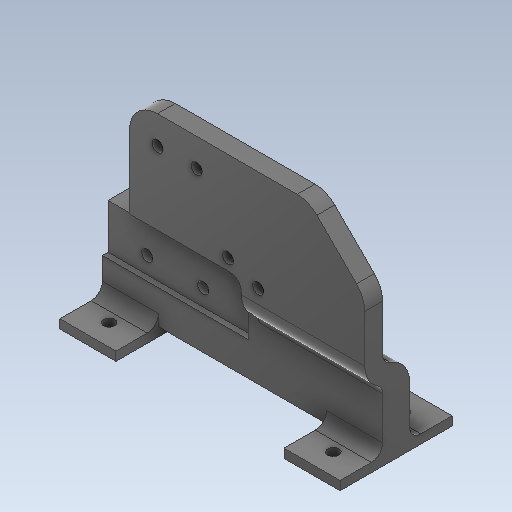
# Autodesk Inventor part: body
Saved by Autodesk Inventor 2020.3 (Build 243373000, 373)
## iProperties
Created: 2021-06-19
Part Number: body
Material: Steel, Mild
Document SubType Name: Modeling
Designer: 0x6f736f646f
Density: 7.85 g/cm^3
Appearance: Smooth - Black
Mass: 6199.14 g
Surface Area: 1192.64 cm^2
Volume: 789.699 cm^3
Author: 0x6f736f646f
Autodesk Inventor part; units mm, degrees
ref_plane "YZ Plane" through (0, 0, 0) normal (1, 0, 0) x (0, 1, 0)
sketch "Sketch1" plane through (0, 0, 0) normal (1, 0, 0) x (0, 1, 0)
  line L0 (0, 0) -> (110, 0)
  line L1 (110, 0) -> (110, -15.875)
  line L2 (110, -15.875) -> (0, -15.875)
  line L3 (0, -15.875) -> (0, -40)
  line L4 (0, -40) -> (-15.875, -40)
  line L5 (-15.875, -40) -> (-70, -40)
  line L6 (-70, -40) -> (-70, -15.875)
  line L7 (-70, -15.875) -> (-15.875, -15.875)
  line L8 (-15.875, -15.875) -> (-15.875, 0)
  line L9 (-15.875, 0) -> (0, 0)
  dimension "d1" = 15.875
  dimension "d2" = 40
  dimension "d3" = 70
  dimension "d4" = 180
  dimension "d5" = 15.875
  constraints: 20 end point, 9 perpendicular, 4 point on line, 1 horizontal
  measures "d1" distance of L0.end L1.end
  measures "d2" distance between parallel lines of L5 L0
  measures "d3" distance between parallel lines of L6 L3
  measures "d4" distance between parallel lines of L6 L1
  measures "d5" distance between parallel lines of L3 L8
extrude "Extrusion1" add sketch "Sketch1" along normal blind 250
sketch "Sketch2" plane through (250, 0, 0) normal (1, 0, 0) x (0, 0, -1)
  line L0 (15.875, -15.875) -> (15.875, -70) projected
  line L1 (15.875, -70) -> (-22.0625, -70)
  line L2 (-22.0625, -70) -> (-22.0625, -77.9375)
  line L3 (-22.0625, -77.9375) -> (77.9375, -77.9375)
  line L4 (77.9375, -77.9375) -> (77.9375, -70)
  line L5 (15.875, -70) -> (40, -70) projected
  line L6 (77.9375, -70) -> (40, -70)
  line L7 (40, -70) -> (15.875, -70)
  point P0 (0, 0)
  dimension "d8" = 100
  dimension "d9" = 7.9375
  constraints: 12 end point, 4 perpendicular, 2 collinear, 1 horizontal, 1 point on line
  measures "d8" distance of L2.end L3.end
  measures "d9" distance between parallel lines of L3 L6
extrude "Extrusion2" add sketch "Sketch2" against normal blind 50
sketch "Sketch3" plane through (250, -70, -40) normal (0, 1, 0) x (1, 0, 0)
  circle A0 centre (-25, 18.9688) radius 5
  line L0 (-50, 0) -> (-50, 37.9375) projected
  line L1 (-50, 18.9688) -> (0, 18.9688)
  line L2 (0, 37.9375) -> (0, 0) projected
  point P0 (-250, -40)
  point P1 (-25, 18.9688)
  dimension "d12" = 10
  dimension "d13" = 25
  constraints: 3 midpoint, 2 end point, 1 centre point, 1 coincident
  measures "d12" diameter of A0
  measures "d13" distance from line of L2 A0.centre
extrude "Extrusion3" cut sketch "Sketch3" against normal through all
ref_plane "Work Plane1" through (0, -70, -27.9375) normal (0, 0, 1) x (1, 0, 0)
mirror "Mirror1" about plane through (0, -70, -27.9375) normal (0, 0, 1) of "Extrusion3"
fillet "Fillet1" radius 10 2 edges at (225, -70, -40) (225, -70, -15.875)
ref_plane "Work Plane2" through (125, 0, 0) normal (1, 0, 0) x (0, 0, -1)
mirror "Mirror2" about plane through (125, 0, 0) normal (1, 0, 0) of "Extrusion2", "Extrusion3", "Mirror1", "Fillet1"
sketch "Sketch6" plane through (0, 0, -15.875) normal (0, 0, -1) x (-1, 0, 0)
  line L0 (0, 0) -> (-250, 0) projected
  line L1 (0, 0) -> (-140, 0)
  line L2 (-140, 0) -> (-140, 20)
  line L3 (-140, 20) -> (-40, 20)
  line L4 (-40, 20) -> (-40, 110)
  line L5 (0, 110) -> (-250, 110) projected
  line L6 (-40, 110) -> (0, 110)
  line L7 (0, 0) -> (0, 110) projected
  line L8 (0, 110) -> (0, 0)
  line L9 (-250, 110) -> (-250, 60)
  line L10 (-250, 0) -> (-250, 110) projected
  line L11 (-250, 60) -> (-200, 110)
  line L12 (-200, 110) -> (-250, 110)
  dimension "d28" = 140
  dimension "d29" = 20
  dimension "d30" = 40
  dimension "d33" = 50
  dimension "d34" = 45
  constraints: 18 end point, 4 point on line, 2 collinear, 2 perpendicular, 1 vertical
  measures "d28" distance between parallel lines of L7 L2
  measures "d29" distance between parallel lines of L0 L3
  measures "d30" distance between parallel lines of L7 L4
  measures "d33" distance of L5.end L9.end
  measures "d34" angle of L11 L9
extrude "Extrusion6" cut sketch "Sketch6" against normal through all contours L0 L2 L3 L4 L5 L7 | L9 L5 L11
fillet "Fillet4" radius 25 3 edges at (40, 110, -7.9375) (200, 110, -7.9375) (250, 60, -7.9375)
sketch "Sketch7" plane through (250, 0, -40) normal (0, 0, -1) x (-1, 0, 0)
  circle A0 centre (185, 85) radius 5
  circle A1 centre (150, 85) radius 5
  circle A2 centre (122, 30) radius 5
  circle A3 centre (95, 20) radius 5
  circle A4 centre (165, -25) radius 5
  circle A5 centre (215, -25) radius 5
  line L0 (210, 20) -> (210, 85) projected
  line L1 (110, 0) -> (110, 20) projected
  line L2 (250, 0) -> (0, 0) projected
  line L3 (110, 20) -> (210, 20) projected
  line L4 (250, -60) -> (250, 0) projected
  arc A6 (210, 85) -> (185, 110) centre (185, 85) ccw projected
  dimension "d36" = 35
  dimension "d37" = 88
  dimension "d38" = 15
  dimension "d39" = 25
  dimension "d40" = 10
  dimension "d41" = 50
  dimension "d42" = 35
  dimension "d43" = 10
  constraints: 6 centre point, 5 equal radius, 2 horizontal alignment, 1 concentric, 1 point on line
  measures "d36" distance of A0.centre A1.centre
  measures "d37" distance from line of L0 A2.centre
  measures "d38" distance from line of L1 A3.centre
  measures "d39" distance from line of L2 A5.centre
  measures "d40" distance from line of L3 A2.centre
  measures "d41" distance of A5.centre A4.centre
  measures "d42" distance from line of L4 A5.centre
  measures "d43" diameter of A0
extrude "Extrusion7" cut sketch "Sketch7" against normal through all
sketch "Sketch8" plane through (0, 0, 0) normal (-1, 0, 0) x (0, 0, 1)
  line L0 (0, 0) -> (-40, 0)
  line L1 (-40, 0) -> (-40, -40)
  line L2 (-40, -60) -> (-40, 0) projected
  line L3 (-40, -40) -> (-15.875, -40)
  line L4 (-15.875, -15.875) -> (-15.875, -60) projected
  line L5 (-15.875, -40) -> (-15.875, -15.875)
  line L6 (0, -15.875) -> (-15.875, -15.875) projected
  line L7 (-15.875, -15.875) -> (0, -15.875)
  line L8 (0, -15.875) -> (0, 0)
  dimension "d46" = 40
  constraints: 12 end point, 3 perpendicular, 2 point on line, 1 horizontal, 1 vertical
  measures "d46" distance between parallel lines of L3 L0
extrude "Extrusion8" cut sketch "Sketch8" against normal blind 170
fillet "Fillet5" radius 10 1 edges at (140, 20, -7.9375)
fillet "Fillet6" radius 25 1 edges at (210, 0, -40)
fillet "Fillet7" radius 10 1 edges at (210, 0, -15.875)
sketch "Sketch9" plane through (170, 0, 0) normal (-1, 0, 0) x (0, 0, 1)
  line L0 (0, 0) -> (0, -15.875) projected
  line L1 (0, -15.875) -> (-15.875, -15.875) projected
  line L2 (0, -15.875) -> (-15.875, -15.875)
  line L3 (-15.875, -15.875) -> (-15.875, -40.0049)
  line L4 (-15.875, -40.0049) -> (-40, -40.0049)
  line L5 (-40, -60) -> (-40, -24.9847) projected
  line L6 (-40, -40.0049) -> (-40, 0)
  line L7 (-40, 0) -> (0, 0)
  line L8 (0, 0) -> (0, -15.875)
  constraints: 12 end point, 4 perpendicular, 1 horizontal, 1 point on line, 1 vertical
extrude "Extrusion9" add sketch "Sketch9" along normal up to surface (30 mm away)
sketch "Sketch10" plane through (140, -15.875, -15.875) normal (-1, 0, 0) x (0, 0, 1)
  line L0 (0, -24.125) -> (0, 0) projected
  line L1 (-24.125, 15.875) -> (0, 15.875)
  line L2 (0, 15.875) -> (0, -24.125)
  line L3 (0, -24.125) -> (-24.125, -24.125)
  line L4 (-24.125, -24.125) -> (-24.125, 15.875)
  line L5 (-24.125, -44.125) -> (-24.125, -24.125) projected
  point P0 (15.875, 15.875)
  point P1 (0, 0)
  point P2 (-24.125, -34.125)
  dimension "d58" = 40
  constraints: 8 end point, 2 parallel, 1 horizontal, 1 midpoint, 1 perpendicular, 1 point on line
  measures "d58" distance between parallel lines of L3 L1
extrude "Extrusion10" add sketch "Sketch10" along normal up to surface (140 mm away)
fillet "Fillet8" radius 25 1 edges at (195, -15.875, 0)
fillet "Fillet9" radius 10 1 edges at (195, -15.875, -15.875)
sketch "Sketch11" plane through (0, 0, 0) normal (-1, 0, 0) x (0, 0, 1)
  line L0 (-15.875, 8.2829) -> (-15.875, 0) projected
  line L1 (-15.875, 0) -> (-20.875, 0)
  line L2 (-20.875, 0) -> (-20.875, -40)
  line L3 (-20.875, -40) -> (-15.875, -40)
  line L4 (-15.875, -40) -> (-15.875, 0)
  point P0 (0, 0)
  dimension "d59" = 5
  dimension "d60" = 40
  constraints: 8 end point, 2 parallel, 1 horizontal, 1 perpendicular
  measures "d59" distance of L3.end L2.end
  measures "d60" distance of L2.end L1.end
extrude "Extrusion11" cut sketch "Sketch11" against normal blind 130
sketch "Sketch12" plane through (250, -60, -40) normal (0, 0, -1) x (-1, 0, 0)
  circle A0 centre (215, 35) radius 5
  circle A1 centre (165, 35) radius 5
  line L0 (80, 60) -> (250, 60) projected
  line L1 (250, 0) -> (250, 60) projected
  dimension "d63" = 25
  dimension "d64" = 50
  dimension "d65" = 10
  dimension "d66" = 35
  constraints: 2 centre point, 1 equal radius, 1 horizontal alignment
  measures "d63" distance from line of L0 A0.centre
  measures "d64" distance of A1.centre A0.centre
  measures "d65" diameter of A0
  measures "d66" distance from line of L1 A0.centre
extrude "Extrusion12" cut sketch "Sketch12" against normal through all
body "Solid1"
